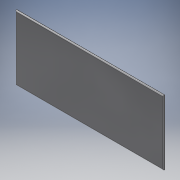
# Autodesk Inventor part: Emblem
Saved by Autodesk Inventor 2018 (Build 220112000, 112)
## iProperties
Created: 2019-05-03
Part Number: Emblem
Material: Aluminum 6061-AHC
Document SubType Name: Modeling
Designer: thatg
Density: 2.7 g/cm^3
Appearance: Aluminum - Dark
Author: thatg
Autodesk Inventor part; units mm, degrees
ref_plane "YZ Plane" through (0, 0, 0) normal (1, 0, 0) x (0, 1, 0)
ref_plane "XZ Plane" through (0, 0, 0) normal (0, 1, 0) x (-1, 0, 0)
ref_plane "XY Plane" through (0, 0, 0) normal (0, 0, 1) x (1, 0, 0)
sketch "Sketch1" plane through (0, 0, 0) normal (0, 0, 1) x (1, 0, 0)
  line L0 (-7.9649, -3.4925) -> (-7.9649, 3.4925) projected
  line L1 (7.9649, -3.4925) -> (-7.9649, -3.4925) projected
  line L2 (7.9649, 3.4925) -> (7.9649, -3.4925) projected
  line L3 (-7.9649, 3.4925) -> (7.9649, 3.4925) projected
  point P0 (0, 0)
extrude "Extrusion1" add sketch "Sketch1" along normal blind 0.0254
sketch "Sketch2" plane through (0, 0, 0.0254) normal (0, 0, 1) x (1, 0, 0)
  line L0 (-7.9649, 3.4925) -> (-7.9649, -3.4925) projected
  line L1 (-7.9649, -3.4925) -> (7.9649, -3.4925) projected
  line L2 (7.9649, -3.4925) -> (7.9649, 3.4925) projected
  line L3 (7.9649, 3.4925) -> (-7.9649, 3.4925) projected
  point P0 (0, 0)
extrude "Extrusion2" add sketch "Sketch2" along normal blind 0.127
fillet "Fillet1" radius 0.127 4 edges at (0, 3.4925, 0.1524) (7.9649, 0, 0.1524) (0, -3.4925, 0.1524) (-7.9649, 0, 0.1524)
body "Solid1"
